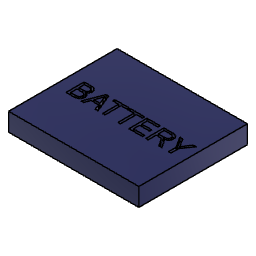
Battery 3.3V v2 (Autodesk Fusion 360 design; units mm, degrees)
Autodesk Fusion 360 part; units mm, degrees
sketch "Sketch1" plane through (0, 0, 0) normal (0, 0, 1) x (1, 0, 0)
  line L0 (0, 0) -> (36, 0)
  line L1 (36, 0) -> (36, 30)
  line L2 (36, 30) -> (0, 30)
  line L3 (0, 30) -> (0, 0)
  dimension "d1" = 36
  dimension "d2" = 30
  constraint horizontal L0
  constraint vertical L1
  constraint horizontal L2
  constraint vertical L3
  constraint coincident L0.start L3.end
  measures "d1" distance of L0.start L0.end
  measures "d2" distance of L0.start L2.end
extrude "Extrude1" add sketch "Sketch1" along normal blind 5
sketch "Sketch2" plane through (0, 0, 5) normal (0, 0, 1) x (-1, 0, 0)
  line L0 (0, -30) -> (0, 0)
  line L1 (0, 0) -> (-36, 0)
  line L2 (-36, 0) -> (-36, -30)
  line L3 (-36, -30) -> (0, -30)
  line L4 (-3.4232, -8.2828) -> (-28.569, -8.2828) construction
  line L5 (-28.569, -8.2828) -> (-28.569, -17.4655) construction
  line L6 (-28.569, -17.4655) -> (-3.4232, -17.4655) construction
  line L7 (-3.4232, -17.4655) -> (-3.4232, -8.2828) construction
  dimension "d5" = 5
  text T0 "BATTERY" font "Arial" height 5 align left top in box 25.1458 x 9.1826 at (-3.4232, -8.2828) x (-1, 0) y (0, -1) spacing 1 kerned
extrude "Extrude2" cut sketch "Sketch2" against normal blind 1 text T0
